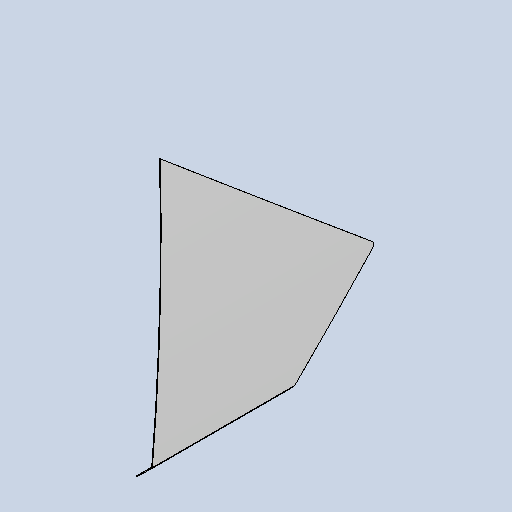
# Autodesk Inventor part: MSC 304 sheet right board face
Saved by Autodesk Inventor 2025 (Build 290162010, 162A)
## iProperties
Created: 2024-04-18
Part Number: MSC 304 sheet right board face
Material: AISI304
Document SubType Name: Sheet Metal
Designer: admin
Stock Number: МОО 304 лист правый борт морда
Mass: 48027.3 g
Surface Area: 40202.8 cm^2
Volume: 6003.41 cm^3
Density: 8 g/cm^3
Sheet Metal Rule: Default_mm
Sheet Metal Width: 980,000 mm
Sheet Metal Length: 1340,712 mm
Sheet Metal Area: 1313897,739 mm^2
Appearance: Default
Flat Pattern Width: 98 cm
Flat Pattern Length: 134.071 cm
Flat Pattern Area: 13139 cm^2
Author: admin
Autodesk Inventor part; units mm, degrees
ref_plane "YZ Plane" through (0, 0, 0) normal (1, 0, 0) x (0, 1, 0)
ref_plane "XZ Plane" through (0, 0, 0) normal (0, 1, 0) x (-1, 0, 0)
ref_plane "XY Plane" through (0, 0, 0) normal (0, 0, 1) x (1, 0, 0)
sketch "Sketch1" plane through (0, 0, 0) normal (0, 0, 1) x (1, 0, 0)
  line L0 (8972.064376, -2416.982713) -> (8972.064376, -2466.982713) construction
  line L1 (0, 47) -> (0, 0) construction
  arc A0 (0.159434, 1.869277) -> (0, 1880) centre (-11009.945504, 940) ccw
  arc A1 (0, 0) -> (0.159434, 1.869277) centre (-11009.945504, 940) ccw construction
  arc A2 (-1.349222, -1.302929) -> (0.159434, 1.869277) centre (-4.822514, 2.29377) ccw
  line L2 (-1.349222, -1.302929) -> (0, 0) construction
  line L3 (-71.93398, -69.465837) -> (-1.349222, -1.302929)
  line L4 (-66.367609, -75.229983) -> (-71.93398, -69.465837) construction
  line L5 (0, 0) -> (0, 1880) construction
  line L6 (0, 0) -> (1.875639, 0) construction
  dimension "d154" = 5
  dimension "d155" = 100
  dimension "d156" = 11050
  dimension "d157" = 136
  dimension "d158" = 1880
  measures "d154" radius of A2
  measures "d155" distance of L1.end L3.start
  measures "d156" radius of A0
  measures "d157" angle of L2 L6
  measures "d158" distance of L1.end L5.end
contour flange "Contour Flange2" sketch "Sketch1" thickness 3 bend radius 3 width 980 along (0, 0, 1) mid plane no both sides no wall seen from (-36.641601, -35.384383, 0) lies toward (0.6946584, -0.7193398, 0) curves L3 A2 A0
bend "Bend2"
corner "Corner2"
sketch "Sketch5" plane through (0, 0, 0) normal (1, 0, 0) x (0, 1, 0)
  line L0 (1.614581, 980) -> (1.614581, 0)
  line L1 (1.614581, 0) -> (1880.255204, 0)
  line L2 (1880.255204, 0) -> (1880.255204, 980)
  line L3 (1.614581, 980) -> (1880.255204, 980)
  line L4 (1.614581, 980) -> (1.614581, 0)
  line L5 (-3.460948, 980) -> (1.614581, 980)
  line L6 (-3.460948, 980) -> (-3.460948, 0)
  line L7 (-3.460948, 0) -> (1.614581, 0)
  line L8 (-3.460948, 980) -> (-3.460948, 0)
  line L9 (-71.623856, 980) -> (-3.460948, 980)
  line L10 (-71.623856, 0) -> (-71.623856, 980)
  line L11 (-71.623856, 0) -> (-3.460948, 0)
  line L12 (1238.605204, 0) -> (416.287565, 980)
  line L13 (395.093292, 980) -> (-71.623856, 588.377813)
  line L14 (395.093292, 0) -> (-71.623856, 391.622187)
  line L15 (416.287565, 0) -> (1238.605204, 980)
  point P0 (0, 0)
  dimension "d161" = 40
  dimension "d162" = 40
  dimension "d163" = 641.65
  dimension "d164" = 641.65
  dimension "d166" = 300
  dimension "d167" = 300
  constraints: 8 end point, 8 point on line, 2 perpendicular
  measures "d161" angle of L2 L15
  measures "d162" angle of L2 L12
  measures "d163" distance of L1.end L12.start
  measures "d164" distance of L2.end L15.end
  measures "d166" distance from line of L9.start L13
  measures "d167" distance from line of L10.start L14
extrude "Extrusion3" cut sketch "Sketch5" along normal through all both and the other way through all contours L14 L1 L0 | L0 L7 L6 L14 | L6 L11 L10 L14 | L3 L2 L1 L12 L15 | L12 L1 L15
sketch "Sketch8" plane through (-1.349222, -1.302929, 980) normal (-0.6946584, 0.7193398, 0) x (0.7193398, 0.6946584, 0)
  line L0 (-61.206441, 25.740843) -> (-79.440024, 25.740843) construction
  line L1 (-79.440024, 25.740843) -> (-79.440024, 162.747026) construction
  line L2 (-79.440024, 162.747026) -> (-61.206441, 162.747026) construction
  line L3 (-61.206441, 162.747026) -> (-61.206441, 25.740843) construction
  point P0 (1.875639, 980)
  constraints: 2 other
mark "Mark5"
equation "\"d36\" = Thickness"
equation "\"d37\" = BendReliefWidth"
equation "\"d38\" = BendReliefDepth"
equation "\"d39\" = MinimumRemnant"
equation "\"d40\" = TransitionRadius"
equation "\"d42\" = BendRadius"
equation "\"d44\" = CornerReliefSize"
equation "\"d45\" = GapSize"
equation "\"d46\" = JacobiRadiusSize"
equation "\"BendRadius\" = Thickness"
equation "\"BendReliefWidth\" = Thickness"
equation "\"BendReliefDepth\" = 0.5 * Thickness"
equation "\"CornerReliefSize\" = 4 * Thickness"
equation "\"MinimumRemnant\" = 2 * Thickness"
equation "\"TransitionRadius\" = BendRadius"
equation "\"JacobiRadiusSize\" = BendRadius"
equation "\"GapSize\" = Thickness"
equation "\"Thickness\" = 3"
body "Solid3"
